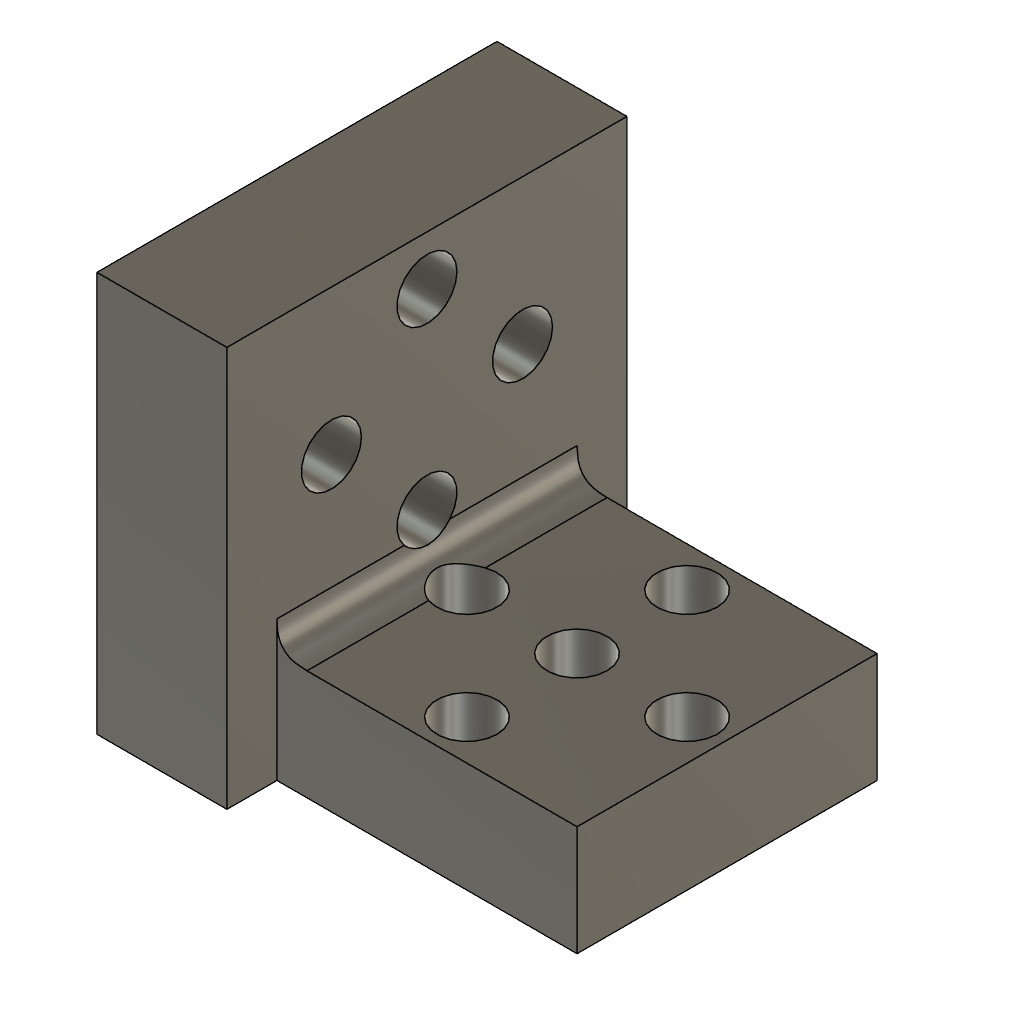
Motor_Mount (Autodesk Fusion 360 design; units mm, degrees)
part number: 2026-09-16-16-56-53-182
Autodesk Fusion 360 part; units mm, degrees
sketch "Sketch1" plane through (0, 0, 0) normal (0, 0, 1) x (1, 0, 0)
  line L0 (0, 0) -> (30, 0)
  line L1 (30, 0) -> (30, 30)
  line L2 (30, 30) -> (0, 30)
  line L3 (0, 30) -> (0, 0)
  dimension "d10" = 30
  dimension "d11" = 30
  constraint horizontal L0
  constraint vertical L1
  constraint horizontal L2
  constraint vertical L3
  constraint coincident L0.start L3.end
  measures "d10" distance of L0.start L0.end
  measures "d11" distance of L0.start L2.end
extrude "Extrude1" add sketch "Sketch1" along normal blind 11
sketch "Sketch2" plane through (0, 0, 0) normal (1, 0, 0) x (0, 1, 0)
  line L0 (-5, 0) -> (35, 0)
  line L1 (35, 0) -> (35, 40)
  line L2 (35, 40) -> (-5, 40)
  line L3 (-5, 40) -> (-5, 0)
  dimension "d14" = 40
  dimension "d15" = 40
  constraint horizontal L0
  constraint vertical L1
  constraint horizontal L2
  constraint vertical L3
  measures "d14" distance of L0.start L0.end
  measures "d15" distance of L0.start L2.end
extrude "Extrude2" add sketch "Sketch2" against normal blind 13
hole "Hole1" at (15, 15, 11) direction (0, 0, -1) diameter 6 depth 15 tip angle 118
sketch "Sketch3" plane through (0, 0, 11) normal (0, 0, 1) x (-1, 0, 0)
  circle A0 centre (-15, -15) radius 3
  line L0 (0, -30) -> (0, 0)
  line L1 (0, 0) -> (-30, 0)
  line L2 (-30, 0) -> (-30, -30)
  line L3 (-30, -30) -> (0, -30)
  circle A1 centre (-15, -15) radius 11
  circle A2 centre (-4, -15) radius 1 construction
  circle A3 centre (-15, -26) radius 0.8867 construction
  circle A4 centre (-26, -15) radius 1 construction
  circle A5 centre (-15, -4) radius 0.9365 construction
  dimension "d23" = 22
  constraint concentric A0 A1
  constraint coincident A1 A2.centre
  constraint coincident A1 A3.centre
  constraint coincident A1 A4.centre
  constraint coincident A1 A5.centre
  measures "d23" diameter of A1
hole "Hole2" at (4, 15, 11) at (15, 26, 11) at (26, 15, 11) at (15, 4, 11) direction (0, 0, -1) diameter 6 end through all
sketch "Sketch4" plane through (0, 0, 0) normal (1, 0, 0) x (0, 1, 0)
  line L0 (30, 11) -> (30, 0)
  line L1 (30, 0) -> (35, 0)
  line L2 (35, 0) -> (35, 40)
  line L3 (35, 40) -> (-5, 40)
  line L4 (-5, 40) -> (-5, 0)
  line L5 (-5, 0) -> (0, 0)
  line L6 (0, 0) -> (0, 11)
  line L7 (0, 11) -> (30, 11)
  line L8 (15, 40) -> (15, 11) construction
  line L9 (15, 25.5) -> (-5, 25.5) construction
  line L10 (15, 25.5) -> (35, 25.5) construction
  circle A0 centre (15, 25.5) radius 9.5525 construction
  circle A1 centre (15, 35.0525) radius 0.9475 construction
  circle A2 centre (24.5525, 25.5) radius 0.7982 construction
  circle A3 centre (15, 15.9475) radius 1.0525 construction
  circle A4 centre (5.4475, 25.5) radius 0.8032 construction
  constraint midpoint L3 L8.start
  constraint midpoint L7 L8.end
  constraint midpoint L8 L9.start
  constraint coincident L4 L9.end
  constraint perpendicular L4 L9
  constraint coincident L2 L10.end
  constraint perpendicular L2 L10
  constraint coincident L9.start L10.start
  constraint coincident A0 A1.centre
  constraint coincident L8 A1.centre
  constraint coincident A0 A2.centre
  constraint coincident L10 A2.centre
  constraint coincident L8 A3.centre
  constraint coincident A0 A3.centre
  constraint coincident A0 A4.centre
  constraint coincident L9 A4.centre
hole "Hole3" at (0, 15, 35.0525) at (0, 24.5525, 25.5) at (0, 15, 15.9475) at (0, 5.4475, 25.5) direction (-1, 0, 0) diameter 6 end through all
fillet "Fillet1" radius 3 tangency weight 1.72216 1 edges at (0, 15, 11)
ref_plane "WorkPlane1" through (15, 15, 7) normal (0, -1, 0) x (1, 0, 0)
sketch "Sketch5" plane through (0, 15, 0) normal (0, -1, 0) x (-1, 0, 0)
equation "b1 = 30 mm"
equation "h1 = 11 mm"
equation "L1 = 30 mm"
equation "b2 = 40 mm"
equation "h2 = 13 mm"
equation "L2 = 40 mm"
equation "hole_wall = 3.4 mm"
equation "hole_motor = 3.4 mm"
equation "hole_shaft = 6 mm"
equation "d10 = b1"
equation "d11 = L1"
equation "d12 = h1"
equation "d14 = b2"
equation "d15 = L2"
equation "d16 = -h2"
equation "d19 = hole_shaft"
